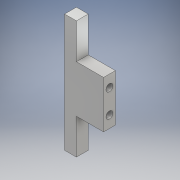
# Autodesk Inventor part: tap_straight
Saved by Autodesk Inventor 2018 (Build 220112000, 112)
## iProperties
Created: 2018-03-14
Part Number: tap_straight
Material: Générique
Document SubType Name: Modeling
Designer: Gregwar
Density: 1 g/cm^3
Appearance: Par défaut
Author: Gregwar
Autodesk Inventor part; units mm, degrees
ref_plane "YZ Plane" through (0, 0, 0) normal (1, 0, 0) x (0, 1, 0)
ref_plane "XZ Plane" through (0, 0, 0) normal (0, 1, 0) x (-1, 0, 0)
ref_plane "XY Plane" through (0, 0, 0) normal (0, 0, 1) x (1, 0, 0)
sketch "Esquisse1" plane through (0, 0, 0) normal (0, 1, 0) x (-1, 0, 0)
  line L0 (0, 0) -> (11.5, 0)
  line L1 (11.5, 0) -> (11.5, -20)
  line L2 (11.5, -20) -> (0, -20)
  line L3 (0, -20) -> (0, 0)
  line L4 (16.5, 15) -> (11.5, 15)
  line L5 (11.5, 15) -> (11.5, -35)
  line L6 (11.5, -35) -> (16.5, -35)
  line L7 (16.5, -35) -> (16.5, 15)
  point P0 (11.5, -10)
  dimension "d0" = 20
  dimension "d1" = 11.5
  dimension "d2" = 5
  dimension "d3" = 50
  constraints: 16 end point, 4 parallel, 2 horizontal, 2 midpoint, 2 perpendicular
  measures "d0" distance of L2.end L0.start
  measures "d1" distance between parallel lines of L3 L5
  measures "d2" distance between parallel lines of L1 L7
  measures "d3" distance of L6.end L4.start
extrude "Extrusion1" add sketch "Esquisse1" along normal blind 5
sketch "Esquisse2" plane through (0, 0, 0) normal (1, 0, 0) x (0, 0, -1)
  line L0 (0, 0) -> (20, 0) construction
  line L1 (20, 0) -> (20, 5) construction
  line L2 (0, 5) -> (20, 5) construction
  line L3 (0, 0) -> (0, 5) construction
  line L4 (0, 0) -> (0, 5) construction
  line L5 (0, 2.5) -> (20, 2.5) construction
  circle A0 centre (5, 2.5) radius 1.5
  line L6 (10, 5) -> (10, 0) construction
  circle A1 centre (15, 2.5) radius 1.5
  dimension "d6" = 3
  dimension "d7" = 10
  constraints: 4 end point, 4 midpoint, 2 centre point, 1 point on line, 1 symmetric about line, 1 other
  measures "d6" diameter of A0
  measures "d7" distance of A1.centre A0.centre
extrude "Extrusion2" cut sketch "Esquisse2" against normal blind 5
